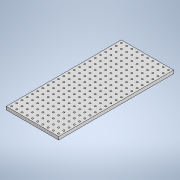
# Autodesk Inventor part: Макетная плата 22
Saved by Autodesk Inventor 2020 (Build 240168000, 168)
## iProperties
Created: 2021-08-09
Part Number: Макетная плата 22
Material: Типовые
Document SubType Name: Modeling
Designer: Антон
Density: 1 g/cm^3
Appearance: По умолчанию
Author: Антон
Autodesk Inventor part; units mm, degrees
ref_plane "YZ Plane" through (0, 0, 0) normal (1, 0, 0) x (0, 1, 0)
ref_plane "XZ Plane" through (0, 0, 0) normal (0, 1, 0) x (-1, 0, 0)
ref_plane "XY Plane" through (0, 0, 0) normal (0, 0, 1) x (1, 0, 0)
sketch "Эскиз1" plane through (0, 0, 0) normal (0, 1, 0) x (-1, 0, 0)
  line L0 (0, 0) -> (25.4, 0)
  line L1 (25.4, 0) -> (25.4, -55.88)
  line L2 (25.4, -55.88) -> (0, -55.88)
  line L3 (0, -55.88) -> (0, 0)
  line L4 (24.13, -1.27) -> (24.13, 0) construction
  line L5 (24.13, -1.27) -> (25.4, -1.27) construction
  line L6 (1.27, -54.61) -> (0, -54.61) construction
  line L7 (1.27, -54.61) -> (1.27, -55.88) construction
  point P0 (24.13, -3.81)
  point P1 (24.13, -6.35)
  point P2 (24.13, -8.89)
  point P3 (24.13, -11.43)
  point P4 (24.13, -13.97)
  point P5 (24.13, -16.51)
  point P6 (24.13, -19.05)
  point P7 (24.13, -21.59)
  point P8 (24.13, -24.13)
  point P9 (24.13, -26.67)
  point P10 (24.13, -29.21)
  point P11 (24.13, -31.75)
  point P12 (24.13, -34.29)
  point P13 (24.13, -36.83)
  point P14 (24.13, -39.37)
  point P15 (24.13, -41.91)
  point P16 (24.13, -44.45)
  point P17 (24.13, -46.99)
  point P18 (24.13, -49.53)
  point P19 (24.13, -52.07)
  point P20 (24.13, -54.61)
  point P21 (21.59, -1.27)
  point P22 (21.59, -3.81)
  point P23 (21.59, -6.35)
  point P24 (21.59, -8.89)
  point P25 (21.59, -11.43)
  point P26 (21.59, -13.97)
  point P27 (21.59, -16.51)
  point P28 (21.59, -19.05)
  point P29 (21.59, -21.59)
  point P30 (21.59, -24.13)
  point P31 (21.59, -26.67)
  point P32 (21.59, -29.21)
  point P33 (21.59, -31.75)
  point P34 (21.59, -34.29)
  point P35 (21.59, -36.83)
  point P36 (21.59, -39.37)
  point P37 (21.59, -41.91)
  point P38 (21.59, -44.45)
  point P39 (21.59, -46.99)
  point P40 (21.59, -49.53)
  point P41 (21.59, -52.07)
  point P42 (21.59, -54.61)
  point P43 (19.05, -1.27)
  point P44 (19.05, -3.81)
  point P45 (19.05, -6.35)
  point P46 (19.05, -8.89)
  point P47 (19.05, -11.43)
  point P48 (19.05, -13.97)
  point P49 (19.05, -16.51)
  point P50 (19.05, -19.05)
  point P51 (19.05, -21.59)
  point P52 (19.05, -24.13)
  point P53 (19.05, -26.67)
  point P54 (19.05, -29.21)
  point P55 (19.05, -31.75)
  point P56 (19.05, -34.29)
  point P57 (19.05, -36.83)
  point P58 (19.05, -39.37)
  point P59 (19.05, -41.91)
  point P60 (19.05, -44.45)
  point P61 (19.05, -46.99)
  point P62 (19.05, -49.53)
  point P63 (19.05, -52.07)
  point P64 (19.05, -54.61)
  point P65 (16.51, -1.27)
  point P66 (16.51, -3.81)
  point P67 (16.51, -6.35)
  point P68 (16.51, -8.89)
  point P69 (16.51, -11.43)
  point P70 (16.51, -13.97)
  point P71 (16.51, -16.51)
  point P72 (16.51, -19.05)
  point P73 (16.51, -21.59)
  point P74 (16.51, -24.13)
  point P75 (16.51, -26.67)
  point P76 (16.51, -29.21)
  point P77 (16.51, -31.75)
  point P78 (16.51, -34.29)
  point P79 (16.51, -36.83)
  point P80 (16.51, -39.37)
  point P81 (16.51, -41.91)
  point P82 (16.51, -44.45)
  point P83 (16.51, -46.99)
  point P84 (16.51, -49.53)
  point P85 (16.51, -52.07)
  point P86 (16.51, -54.61)
  point P87 (13.97, -1.27)
  point P88 (13.97, -3.81)
  point P89 (13.97, -6.35)
  point P90 (13.97, -8.89)
  point P91 (13.97, -11.43)
  point P92 (13.97, -13.97)
  point P93 (13.97, -16.51)
  point P94 (13.97, -19.05)
  point P95 (13.97, -21.59)
  point P96 (13.97, -24.13)
  point P97 (13.97, -26.67)
  point P98 (13.97, -29.21)
  point P99 (13.97, -31.75)
  point P100 (13.97, -34.29)
  point P101 (13.97, -36.83)
  point P102 (13.97, -39.37)
  point P103 (13.97, -41.91)
  point P104 (13.97, -44.45)
  point P105 (13.97, -46.99)
  point P106 (13.97, -49.53)
  point P107 (13.97, -52.07)
  point P108 (13.97, -54.61)
  point P109 (11.43, -1.27)
  point P110 (11.43, -3.81)
  point P111 (11.43, -6.35)
  point P112 (11.43, -8.89)
  point P113 (11.43, -11.43)
  point P114 (11.43, -13.97)
  point P115 (11.43, -16.51)
  point P116 (11.43, -19.05)
  point P117 (11.43, -21.59)
  point P118 (11.43, -24.13)
  point P119 (11.43, -26.67)
  point P120 (11.43, -29.21)
  point P121 (11.43, -31.75)
  point P122 (11.43, -34.29)
  point P123 (11.43, -36.83)
  point P124 (11.43, -39.37)
  point P125 (11.43, -41.91)
  point P126 (11.43, -44.45)
  point P127 (11.43, -46.99)
  point P128 (11.43, -49.53)
  point P129 (11.43, -52.07)
  point P130 (11.43, -54.61)
  point P131 (8.89, -1.27)
  point P132 (8.89, -3.81)
  point P133 (8.89, -6.35)
  point P134 (8.89, -8.89)
  point P135 (8.89, -11.43)
  point P136 (8.89, -13.97)
  point P137 (8.89, -16.51)
  point P138 (8.89, -19.05)
  point P139 (8.89, -21.59)
  point P140 (8.89, -24.13)
  point P141 (8.89, -26.67)
  point P142 (8.89, -29.21)
  point P143 (8.89, -31.75)
  point P144 (8.89, -34.29)
  point P145 (8.89, -36.83)
  point P146 (8.89, -39.37)
  point P147 (8.89, -41.91)
  point P148 (8.89, -44.45)
  point P149 (8.89, -46.99)
  point P150 (8.89, -49.53)
  point P151 (8.89, -52.07)
  point P152 (8.89, -54.61)
  point P153 (6.35, -1.27)
  point P154 (6.35, -3.81)
  point P155 (6.35, -6.35)
  point P156 (6.35, -8.89)
  point P157 (6.35, -11.43)
  point P158 (6.35, -13.97)
  point P159 (6.35, -16.51)
  point P160 (6.35, -19.05)
  point P161 (6.35, -21.59)
  point P162 (6.35, -24.13)
  point P163 (6.35, -26.67)
  point P164 (6.35, -29.21)
  point P165 (6.35, -31.75)
  point P166 (6.35, -34.29)
  point P167 (6.35, -36.83)
  point P168 (6.35, -39.37)
  point P169 (6.35, -41.91)
  point P170 (6.35, -44.45)
  point P171 (6.35, -46.99)
  point P172 (6.35, -49.53)
  point P173 (6.35, -52.07)
  point P174 (6.35, -54.61)
  point P175 (3.81, -1.27)
  point P176 (3.81, -3.81)
  point P177 (3.81, -6.35)
  point P178 (3.81, -8.89)
  point P179 (3.81, -11.43)
  point P180 (3.81, -13.97)
  point P181 (3.81, -16.51)
  point P182 (3.81, -19.05)
  point P183 (3.81, -21.59)
  point P184 (3.81, -24.13)
  point P185 (3.81, -26.67)
  point P186 (3.81, -29.21)
  point P187 (3.81, -31.75)
  point P188 (3.81, -34.29)
  point P189 (3.81, -36.83)
  point P190 (3.81, -39.37)
  point P191 (3.81, -41.91)
  point P192 (3.81, -44.45)
  point P193 (3.81, -46.99)
  point P194 (3.81, -49.53)
  point P195 (3.81, -52.07)
  point P196 (3.81, -54.61)
  point P197 (1.27, -1.27)
  point P198 (1.27, -3.81)
  point P199 (1.27, -6.35)
  dimension "d2" = 2.54
  dimension "d5" = 2.54
  dimension "d8" = 1.27
  constraints: 16 end point, 7 perpendicular, 4 point on line, 2 horizontal, 2 parallel, 2 vertical, 219 other
  measures "d2" distance of L4.start point (24.13, -3.81)
  measures "d5" distance of L4.start point (21.59, -1.27)
  measures "d8" distance from line of L1 L4.start
extrude "Выдавливание1" add sketch "Эскиз1" along normal blind 1.5
hole "Отверстие1" at (-24.13, 0, -1.27) at (-24.13, 0, -3.81) at (-24.13, 0, -6.35) at (-24.13, 0, -8.89) at (-24.13, 0, -11.43) at (-24.13, 0, -13.97) at (-24.13, 0, -16.51) at (-24.13, 0, -19.05) at (-24.13, 0, -21.59) at (-24.13, 0, -24.13) at (-24.13, 0, -26.67) at (-24.13, 0, -29.21) at (-24.13, 0, -31.75) at (-24.13, 0, -34.29) at (-24.13, 0, -36.83) at (-24.13, 0, -39.37) at (-24.13, 0, -41.91) at (-24.13, 0, -44.45) at (-24.13, 0, -46.99) at (-24.13, 0, -49.53) at (-24.13, 0, -52.07) at (-24.13, 0, -54.61) at (-21.59, 0, -1.27) at (-21.59, 0, -3.81) at (-21.59, 0, -6.35) at (-21.59, 0, -8.89) at (-21.59, 0, -11.43) at (-21.59, 0, -13.97) at (-21.59, 0, -16.51) at (-21.59, 0, -19.05) at (-21.59, 0, -21.59) at (-21.59, 0, -24.13) at (-21.59, 0, -26.67) at (-21.59, 0, -29.21) at (-21.59, 0, -31.75) at (-21.59, 0, -34.29) at (-21.59, 0, -36.83) at (-21.59, 0, -39.37) at (-21.59, 0, -41.91) at (-21.59, 0, -44.45) at (-21.59, 0, -46.99) at (-21.59, 0, -49.53) at (-21.59, 0, -52.07) at (-21.59, 0, -54.61) at (-19.05, 0, -1.27) at (-19.05, 0, -3.81) at (-19.05, 0, -6.35) at (-19.05, 0, -8.89) at (-19.05, 0, -11.43) at (-19.05, 0, -13.97) direction (0, 1, 0) diameter 0.8 end through all and at (-19.05, 0, -16.51) (-19.05, 0, -19.05) (-19.05, 0, -21.59) (-19.05, 0, -24.13) (-19.05, 0, -26.67) (-19.05, 0, -29.21) (-19.05, 0, -31.75) (-19.05, 0, -34.29) (-19.05, 0, -36.83) (-19.05, 0, -39.37) (-19.05, 0, -41.91) (-19.05, 0, -44.45) (-19.05, 0, -46.99) (-19.05, 0, -49.53) (-19.05, 0, -52.07) (-19.05, 0, -54.61) (-16.51, 0, -1.27) (-16.51, 0, -3.81) (-16.51, 0, -6.35) (-16.51, 0, -8.89) (-16.51, 0, -11.43) (-16.51, 0, -13.97) (-16.51, 0, -16.51) (-16.51, 0, -19.05) (-16.51, 0, -21.59) (-16.51, 0, -24.13) (-16.51, 0, -26.67) (-16.51, 0, -29.21) (-16.51, 0, -31.75) (-16.51, 0, -34.29) (-16.51, 0, -36.83) (-16.51, 0, -39.37) (-16.51, 0, -41.91) (-16.51, 0, -44.45) (-16.51, 0, -46.99) (-16.51, 0, -49.53) (-16.51, 0, -52.07) (-16.51, 0, -54.61) (-13.97, 0, -1.27) (-13.97, 0, -3.81) (-13.97, 0, -6.35) (-13.97, 0, -8.89) (-13.97, 0, -11.43) (-13.97, 0, -13.97) (-13.97, 0, -16.51) (-13.97, 0, -19.05) (-13.97, 0, -21.59) (-13.97, 0, -24.13) (-13.97, 0, -26.67) (-13.97, 0, -29.21) (-13.97, 0, -31.75) (-13.97, 0, -34.29) (-13.97, 0, -36.83) (-13.97, 0, -39.37) (-13.97, 0, -41.91) (-13.97, 0, -44.45) (-13.97, 0, -46.99) (-13.97, 0, -49.53) (-13.97, 0, -52.07) (-13.97, 0, -54.61) (-11.43, 0, -1.27) (-11.43, 0, -3.81) (-11.43, 0, -6.35) (-11.43, 0, -8.89) (-11.43, 0, -11.43) (-11.43, 0, -13.97) (-11.43, 0, -16.51) (-11.43, 0, -19.05) (-11.43, 0, -21.59) (-11.43, 0, -24.13) (-11.43, 0, -26.67) (-11.43, 0, -29.21) (-11.43, 0, -31.75) (-11.43, 0, -34.29) (-11.43, 0, -36.83) (-11.43, 0, -39.37) (-11.43, 0, -41.91) (-11.43, 0, -44.45) (-11.43, 0, -46.99) (-11.43, 0, -49.53) (-11.43, 0, -52.07) (-11.43, 0, -54.61) (-8.89, 0, -1.27) (-8.89, 0, -3.81) (-8.89, 0, -6.35) (-8.89, 0, -8.89) (-8.89, 0, -11.43) (-8.89, 0, -13.97) (-8.89, 0, -16.51) (-8.89, 0, -19.05) (-8.89, 0, -21.59) (-8.89, 0, -24.13) (-8.89, 0, -26.67) (-8.89, 0, -29.21) (-8.89, 0, -31.75) (-8.89, 0, -34.29) (-8.89, 0, -36.83) (-8.89, 0, -39.37) (-8.89, 0, -41.91) (-8.89, 0, -44.45) (-8.89, 0, -46.99) (-8.89, 0, -49.53) (-8.89, 0, -52.07) (-8.89, 0, -54.61) (-6.35, 0, -1.27) (-6.35, 0, -3.81) (-6.35, 0, -6.35) (-6.35, 0, -8.89) (-6.35, 0, -11.43) (-6.35, 0, -13.97) (-6.35, 0, -16.51) (-6.35, 0, -19.05) (-6.35, 0, -21.59) (-6.35, 0, -24.13) (-6.35, 0, -26.67) (-6.35, 0, -29.21) (-6.35, 0, -31.75) (-6.35, 0, -34.29) (-6.35, 0, -36.83) (-6.35, 0, -39.37) (-6.35, 0, -41.91) (-6.35, 0, -44.45) (-6.35, 0, -46.99) (-6.35, 0, -49.53) (-6.35, 0, -52.07) (-6.35, 0, -54.61) (-3.81, 0, -1.27) (-3.81, 0, -3.81) (-3.81, 0, -6.35) (-3.81, 0, -8.89) (-3.81, 0, -11.43) (-3.81, 0, -13.97) (-3.81, 0, -16.51) (-3.81, 0, -19.05) (-3.81, 0, -21.59) (-3.81, 0, -24.13) (-3.81, 0, -26.67) (-3.81, 0, -29.21) (-3.81, 0, -31.75) (-3.81, 0, -34.29) (-3.81, 0, -36.83) (-3.81, 0, -39.37) (-3.81, 0, -41.91) (-3.81, 0, -44.45) (-3.81, 0, -46.99) (-3.81, 0, -49.53) (-3.81, 0, -52.07) (-3.81, 0, -54.61) (-1.27, 0, -1.27) (-1.27, 0, -3.81) (-1.27, 0, -6.35) (-1.27, 0, -8.89) (-1.27, 0, -11.43) (-1.27, 0, -13.97) (-1.27, 0, -16.51) (-1.27, 0, -19.05) (-1.27, 0, -21.59) (-1.27, 0, -24.13) (-1.27, 0, -26.67) (-1.27, 0, -29.21) (-1.27, 0, -31.75) (-1.27, 0, -34.29) (-1.27, 0, -36.83) (-1.27, 0, -39.37) (-1.27, 0, -41.91) (-1.27, 0, -44.45) (-1.27, 0, -46.99) (-1.27, 0, -49.53) (-1.27, 0, -52.07) (-1.27, 0, -54.61)
